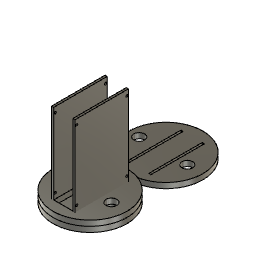
flightcomputerv2 v0 (Autodesk Fusion 360 design; units mm, degrees)
Autodesk Fusion 360 part; units mm, degrees
sketch "Sketch1" plane through (0, 0, 0) normal (0, 0, 1) x (1, 0, 0)
  circle A0 centre (0, 0) radius 34.5
  line L0 (-9, 37) -> (9, 37) construction
  line L1 (9, 37) -> (9, -40) construction
  line L2 (9, -40) -> (-9, -40) construction
  line L3 (-9, -40) -> (-9, 22) construction
  line L4 (-9, 22) -> (-9, 37) construction
  line L5 (41, -25) -> (41, 25) construction
  line L6 (41, 25) -> (-51, 25) construction
  line L7 (-51, 25) -> (-51, -25) construction
  line L8 (-51, -25) -> (41, -25) construction
  line L9 (9, 25) -> (11, 25)
  line L10 (11, 25) -> (11, -25)
  line L11 (9, -25) -> (11, -25)
  line L12 (9, -25) -> (9, 25)
  line L13 (-9, -25) -> (-9, 25)
  line L14 (-9, 25) -> (-11, 25)
  line L15 (-11, -25) -> (-11, 25)
  line L16 (-11, -25) -> (-9, -25)
  line L17 (9, 25) -> (9, 0) construction
  line L18 (-9, 25) -> (9, 25)
  line L19 (9, -25) -> (-9, -25)
  dimension "d1" = 69
  dimension "d2" = 18
  dimension "d3" = 50
  dimension "d4" = 2
  dimension "d5" = 25
  constraint coincident A0.centre origin
  constraint horizontal L0
  constraint perpendicular L0 L1
  constraint perpendicular L1 L2
  constraint perpendicular L2 L3
  constraint parallel L1 L5
  constraint perpendicular L5 L6
  constraint perpendicular L6 L7
  constraint coincident L6 L9.start
  constraint coincident L1 L9.start
  constraint perpendicular L1 L9
  constraint coincident L8 L10.end
  constraint perpendicular L8 L10
  constraint coincident L8 L11.start
  constraint coincident L1 L11.start
  constraint coincident L3 L13.start
  constraint coincident L8 L13.start
  constraint coincident L4 L13.end
  constraint coincident L6 L13.end
  constraint coincident L6 L14.end
  constraint coincident L8 L15.start
  constraint perpendicular L6 L15
  constraint perpendicular L6 L17
  measures "d1" diameter of A0
  measures "d2" distance of L0.start L0.end
  measures "d3" distance of L5.start L5.end
  measures "d4" distance of L9.start L9.end
  measures "d5" distance of L9.start L17.end
extrude "Extrude4" add sketch "Sketch1" along normal blind 85 contours L9 L10 L11 L12 | L13 L14 L15 L16 makes body 1 at (-9, -8.3333, 28.3333) makes body 2 at (9, -8.3333, 28.3333)
extrude "Extrude3" add sketch "Sketch1" along normal blind 10 separate body contours A0 | L9 L10 L11 L12 | L13 L14 L15 L16 makes body 3
extrude "Extrude2" add sketch "Sketch1" along normal blind 5 separate body contours A0 | L9 L10 L11 L12 | L13 L14 L15 L16 makes body 4
extrude "Extrude1" add sketch "Sketch1" along normal blind 5 separate body contours A0 | L9 L10 L11 L12 | L12 L13 L18 L19 | L13 L14 L15 L16 makes body 5
sketch "Sketch2" plane through (11, 0, 0) normal (1, 0, 0) x (0, 1, 0)
  line L0 (-25, 0) -> (25, 0)
  line L1 (25, 0) -> (25, 85)
  line L2 (25, 85) -> (-25, 85)
  line L3 (-25, 85) -> (-25, 0)
  line L4 (30, 15) -> (30, 80) construction
  line L5 (30, 80) -> (-35, 80) construction
  line L6 (-35, 80) -> (-35, 15) construction
  line L7 (-35, 15) -> (30, 15) construction
  line L8 (25, 85) -> (24.5, 85) construction
  line L9 (24.5, 85) -> (24.5, 15) construction
  line L10 (-25, 85) -> (-24.5, 85) construction
  line L11 (-24.5, 85) -> (-24.5, 15) construction
  line L12 (-24.5, 80) -> (-23.5, 80) construction
  circle A0 centre (-23.5, 80) radius 1 construction
  line L13 (24.5, 80) -> (23.5, 80) construction
  circle A1 centre (23.5, 80) radius 1 construction
  line L14 (24.5, 15) -> (23.5, 15) construction
  circle A2 centre (23.5, 15) radius 1 construction
  line L15 (-24.5, 15) -> (-23.5, 15) construction
  circle A3 centre (-23.5, 15) radius 1 construction
  circle A4 centre (-23.5, 15) radius 1
  circle A5 centre (23.5, 15) radius 1
  circle A6 centre (23.5, 80) radius 1
  circle A7 centre (-23.5, 80) radius 1
  dimension "d14" = 65
  dimension "d15" = 0.5
  dimension "d16" = 0.5
  dimension "d17" = 1
  dimension "d18" = 2
  dimension "d19" = 1
  dimension "d20" = 2
  dimension "d21" = 1
  dimension "d22" = 2
  dimension "d23" = 1
  dimension "d24" = 2
  constraint vertical L4
  constraint perpendicular L4 L5
  constraint perpendicular L5 L6
  constraint perpendicular L4 L7
  constraint coincident L1.end L2.start
  constraint horizontal L8
  constraint coincident L7 L9.end
  constraint perpendicular L7 L9
  constraint coincident L2.end L3.start
  constraint horizontal L10
  constraint coincident L7 L11.end
  constraint perpendicular L7 L11
  constraint coincident L5 L12.start
  constraint coincident L11 L12.start
  constraint perpendicular L11 L12
  constraint coincident L12.end A0.centre
  constraint coincident L5 L13.start
  constraint coincident L9 L13.start
  constraint perpendicular L9 L13
  constraint coincident L13.end A1.centre
  constraint perpendicular L9 L14
  constraint coincident L14.end A2.centre
  constraint perpendicular L11 L15
  constraint coincident L15.end A3.centre
  constraint concentric A2 A5
  constraint concentric A1 A6
  measures "d14" distance of L4.start L4.end
  measures "d15" distance of L1.end L8.end
  measures "d16" distance of L2.end L10.end
  measures "d17" distance of L12.start L12.end
  measures "d18" diameter of A0
  measures "d19" distance of L13.start L13.end
  measures "d20" diameter of A1
  measures "d21" distance of L9.end L14.end
  measures "d22" diameter of A2
  measures "d23" distance of L11.end L15.end
  measures "d24" diameter of A3
extrude "Extrude5" cut sketch "Sketch2" against normal blind 40 contours A4 | A5 | A6 | A7 bodies 1 2
move_body "Move1" bodies 1 5 4 3 2 to x (1, 0, 0) y (0, 1, 0) z (0, 0, 1) at (0, -71, 0)
sketch "Sketch3" plane through (0, 0, 0) normal (0, 0, 1) x (1, 0, 0)
  circle A0 centre (0, 0) radius 34.5
  line L0 (40, -25) -> (40, 25) construction
  line L1 (40, 25) -> (-40, 25) construction
  line L2 (-40, 25) -> (-40, -25) construction
  line L3 (-40, -25) -> (40, -25) construction
  line L4 (-9, 40) -> (9, 40) construction
  line L5 (-9, 40) -> (-9, -30) construction
  line L6 (-9, -30) -> (9, -30) construction
  line L7 (9, -30) -> (9, 40) construction
  line L8 (9, 25) -> (11, 25) construction
  line L9 (11, 25) -> (11, -25) construction
  line L10 (-9, 25) -> (-11, 25) construction
  line L11 (-9, 25) -> (-11, 25)
  line L12 (-11, 25) -> (-11, -25)
  line L13 (-11, -25) -> (-9, -25)
  line L14 (-9, -25) -> (-9, 25)
  line L15 (9, 25) -> (11, 25)
  line L16 (11, 25) -> (11, -25)
  line L17 (11, -25) -> (9, -25)
  line L18 (9, -25) -> (9, 25)
  circle A1 centre (-25, 0) radius 5
  circle A2 centre (20, 0) radius 5
  dimension "d27" = 69
  dimension "d28" = 50
  dimension "d29" = 18
  dimension "d30" = 18
  dimension "d31" = 2
  dimension "d32" = 2
  constraint coincident A0.centre origin
  constraint vertical L0
  constraint perpendicular L0 L1
  constraint perpendicular L1 L2
  constraint perpendicular L0 L3
  constraint perpendicular L0 L4
  constraint perpendicular L4 L5
  constraint perpendicular L5 L6
  constraint coincident L7 L8.start
  constraint coincident L1 L8.start
  constraint perpendicular L7 L8
  constraint coincident L3 L9.end
  constraint perpendicular L3 L9
  constraint coincident L5 L10.start
  constraint coincident L1 L10.start
  constraint perpendicular L5 L10
  constraint coincident L3 L12.end
  constraint perpendicular L3 L12
  constraint coincident L3 L13.end
  constraint coincident L5 L13.end
  constraint coincident L7 L17.end
  constraint coincident L3 L17.end
  constraint perpendicular L7 L17
  measures "d27" diameter of A0
  measures "d28" distance of L0.start L0.end
  measures "d29" distance of L4.start L4.end
  measures "d30" distance of L5.end L6.end
  measures "d31" distance of L8.start L8.end
  measures "d32" distance of L10.start L10.end
extrude "Extrude6" add sketch "Sketch3" along normal blind 5 separate body makes body 6
sketch "Sketch4" plane through (0, 0, 10) normal (0, 0, 1) x (-1, 0, 0)
  line L0 (-9, 46) -> (-9, 96)
  line L1 (-9, 96) -> (9, 96)
  line L2 (9, 96) -> (9, 46)
  line L3 (9, 46) -> (-9, 46)
  circle A0 centre (0, 71) radius 34.5
  circle A1 centre (0, 71) radius 34.5 construction
  line L4 (0, 35) -> (0, 110) construction
  line L5 (0, 71) -> (-52.4264, 71) construction
  line L6 (-52.4264, 71) -> (66.3943, 71) construction
  line L7 (25, 105) -> (25, 35) construction
  line L8 (25, 35) -> (20, 35) construction
  line L9 (-20, 110) -> (-20, 35) construction
  circle A2 centre (-20, 71) radius 5
  circle A3 centre (25, 71) radius 5
  dimension "d35" = 10
  dimension "d36" = 10
  constraint concentric A0 A1
  constraint vertical L4
  constraint coincident A0.centre A1.centre
  constraint perpendicular L4 L5
  constraint perpendicular L2 L6
  constraint perpendicular L5 L7
  constraint perpendicular L7 L8
  constraint perpendicular L5 L9
  constraint coincident L9 A2.centre
  constraint coincident L5 A2.centre
  constraint coincident L7 A3.centre
  constraint coincident L6 A3.centre
  measures "d35" diameter of A2
  measures "d36" diameter of A3
extrude "Extrude7" cut sketch "Sketch4" against normal blind 20 contours A2 | A3 bodies 3 4 5
